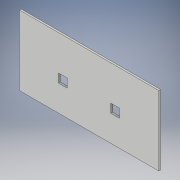
# Autodesk Inventor part: model 1 window board
Saved by Autodesk Inventor 2017 (Build 210142000, 142)
## iProperties
Created: 2017-06-12
Part Number: model 1 window board
Material: Generic
Document SubType Name: Modeling
Designer: cas7
Density: 1 g/cm^3
Appearance: Default
Author: cas7
Autodesk Inventor part; units mm, degrees
ref_plane "YZ Plane" through (0, 0, 0) normal (1, 0, 0) x (0, 1, 0)
ref_plane "XZ Plane" through (0, 0, 0) normal (0, 1, 0) x (-1, 0, 0)
ref_plane "XY Plane" through (0, 0, 0) normal (0, 0, 1) x (1, 0, 0)
sketch "Sketch1" plane through (0, 0, 0) normal (0, 0, 1) x (1, 0, 0)
  line L0 (0, 0) -> (1219.2, 0)
  line L1 (1219.2, 0) -> (1219.2, 609.6)
  line L2 (1219.2, 609.6) -> (0, 609.6)
  line L3 (0, 609.6) -> (0, 0)
  dimension "d0" = 1219.2
  dimension "d1" = 609.6
  constraints: 8 end point, 2 parallel, 1 horizontal, 1 perpendicular
  measures "d0" distance of L2.end L1.end
  measures "d1" distance of L1.end L0.end
extrude "Extrusion1" add sketch "Sketch1" along normal blind 15.875
sketch "Sketch2" plane through (0, 0, 15.875) normal (0, 0, 1) x (1, 0, 0)
  line L0 (342.9, 228.6) -> (419.1, 228.6)
  line L1 (419.1, 228.6) -> (419.1, 304.8)
  line L2 (419.1, 304.8) -> (342.9, 304.29)
  line L3 (342.9, 304.29) -> (342.9, 228.6)
  line L4 (876.3, 228.6) -> (876.3, 304.8)
  line L5 (876.3, 304.8) -> (800.1, 304.8)
  line L6 (800.1, 304.8) -> (800.1, 228.6)
  line L7 (800.1, 228.6) -> (876.3, 228.6)
  dimension "d13" = 76.2
  dimension "d15" = 76.2
  dimension "d16" = 76.2
  dimension "d17" = 76.2
  constraints: 16 end point, 3 perpendicular
  measures "d13" distance of L0.end L1.end
  measures "d15" distance of L4.start L4.end
  measures "d16" distance of L4.end L5.end
  measures "d17" distance of L5.end L6.end
extrude "Extrusion2" cut sketch "Sketch2" against normal blind 15.875
body "Solid1"
